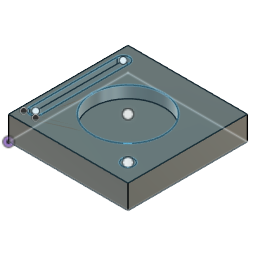
Miliing (Autodesk Fusion 360 design; units mm, degrees)
part number: 2026-06-19-23-17-38-710
Autodesk Fusion 360 part; units mm, degrees
note: some values were not read from the file. Set by a fixed rule: which sketch regions a step uses.
sketch "Sketch1" plane through (0, 0, 0) normal (0, 0, 1) x (1, 0, 0)
  line L0 (0, 0) -> (100, 0)
  line L1 (100, 0) -> (100, 100)
  line L2 (100, 100) -> (0, 100)
  line L3 (0, 100) -> (0, 0)
  dimension "d1" = 100
  dimension "d2" = 100
  constraint horizontal L0
  constraint vertical L1
  constraint horizontal L2
  constraint vertical L3
  constraint coincident L0.start L3.end
  measures "d1" distance of L0.start L2.end
  measures "d2" distance of L0.start L0.end
extrude "Extrude1" add sketch "Sketch1" along normal blind 20
sketch "Sketch2" plane through (0, 0, 20) normal (0, 0, 1) x (-1, 0, 0)
  line L0 (0, -100) -> (0, 0)
  line L1 (0, 0) -> (-100, 0)
  line L2 (-100, 0) -> (-100, -100)
  line L3 (-100, -100) -> (0, -100)
  circle A0 centre (-50, -50) radius 30
extrude "Extrude2" cut sketch "Sketch2" against normal blind 10 contours A0
sketch "Sketch3" plane through (0, 0, 20) normal (0, 0, 1) x (-1, 0, 0)
  circle A0 centre (-50, -50) radius 30
  line L0 (0, -100) -> (0, 0)
  line L1 (0, 0) -> (-100, 0)
  line L2 (-100, 0) -> (-100, -100)
  line L3 (-100, -100) -> (0, -100)
sketch "Sketch4" plane through (0, 0, 20) normal (0, 0, 1) x (-1, 0, 0)
  line L0 (-14, -86.9507) -> (-14, -13.6932)
  line L1 (-4, -13.6932) -> (-4, -86.9507)
  arc A0 (-14, -86.9507) -> (-9, -91.9507) centre (-9, -86.9507) ccw
  arc A1 (-9, -91.9507) -> (-4, -86.9507) centre (-9, -86.9507) ccw
  arc A2 (-9, -8.6932) -> (-14, -13.6932) centre (-9, -13.6932) ccw
  arc A3 (-4, -13.6932) -> (-9, -8.6932) centre (-9, -13.6932) ccw
  point P0 (-14, -8.6932)
  point P1 (-4, -8.6932)
  dimension "d7" = 10
  dimension "d12" = 5
  constraint vertical L0
  constraint vertical L1
  constraint tangent L0 A0
  constraint tangent L1 A1
  constraint equal A0 A1
  constraint coincident A0.end A1.start
  constraint coincident P0 L0
  constraint tangent L0 A2
  constraint equal A0 A2
  constraint coincident P1 L1
  constraint tangent L1 A3
  constraint equal A0 A3
  constraint coincident A2.start A3.end
  measures "d7" distance of P0 P1
  measures "d12" radius of A0
extrude "Extrude3" cut sketch "Sketch4" against normal blind 5
sketch "Sketch5" plane through (0, 0, 0) normal (0, 0, -1) x (1, 0, 0)
  line L0 (0, 0) -> (0, -100)
  line L1 (0, -100) -> (100, -100)
  line L2 (100, -100) -> (100, 0)
  line L3 (100, 0) -> (0, 0)
sketch "Sketch6" plane through (0, 0, 20) normal (0, 0, 1) x (-1, 0, 0)
  circle A0 centre (-85, -15) radius 5
  dimension "d10" = 10
  measures "d10" diameter of A0
extrude "Extrude4" cut sketch "Sketch6" against normal through all
sketch "Sketch7" plane through (0, 0, 20) normal (0, 0, 1) x (-1, 0, 0)
